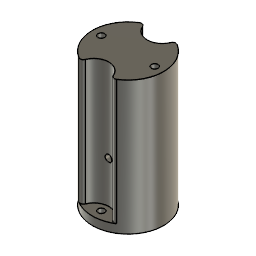
drum (Autodesk Fusion 360 design; units mm, degrees)
part number: 2026-03-23-22-00-02-455
Autodesk Fusion 360 part; units mm, degrees
sketch "Sketch1" plane through (0, 0, 0) normal (0, 0, 1) x (1, 0, 0)
  circle A0 centre (0, 0) radius 10.7
  circle A1 centre (0, 0) radius 4.05
  line L0 (-10, -10) -> (10, 10)
  line L1 (-10, 10) -> (10, -10)
  circle A2 centre (-8, 0) radius 1
  circle A3 centre (-8, 0) radius 2.25
  circle A4 centre (-10.25, 0) radius 4.5
  circle A5 centre (0, -8) radius 1
  circle A6 centre (0, -8) radius 2.25
  circle A7 centre (0, -10.25) radius 4.5
  circle A8 centre (8, 0) radius 2.25
  circle A9 centre (8, 0) radius 1
  circle A10 centre (10.25, 0) radius 4.5
  circle A11 centre (0, 8) radius 1
  circle A12 centre (0, 8) radius 2.25
  circle A13 centre (0, 10.25) radius 4.5
  dimension "d3" = 21.4
  dimension "d4" = 8.1
  dimension "d19" = 2
  constraint concentric A0 A1
  constraint coincident A3 A4.centre
  constraint symmetric L0 A2 A5
  constraint symmetric L0 A3 A6
  constraint symmetric L0 A4 A7
  constraint symmetric L1 A2 A11
  constraint symmetric L1 A3 A12
  constraint symmetric L1 A4 A13
  constraint symmetric L1 A5 A9
  constraint symmetric L1 A6 A8
  constraint symmetric L1 A7 A10
  measures "d3" diameter of A0
  measures "d4" diameter of A1
  measures "d19" diameter of A9
extrude "Extrude1" add sketch "Sketch1" along normal blind 40 contours A8 | A0 A10 | A0 A1 L0 L1 A10 | A0 A1 L0 L1 A13 | A0 A1 L0 L1 A7 | A12 | A0 A13 | A1 L0 L1 | A1 L0 L1 | A6 | A0 A7 | A1 L0 L1 | A1 L0 L1 | A0 A1 L0 L1 A4 | A3 | A0 A4 | A2 | A5 | A9 | A11 picked at (9.1824, 3.0854) picked at (3.1202, 9.1627) picked at (3.1202, -9.1627) picked at (-9.1824, -3.0854)
extrude "Extrude2" cut sketch "Sketch1" along normal blind 2 contours A1 L0 L1 | A1 L0 L1 | A1 L0 L1 | A1 L0 L1
extrude "Extrude3" cut sketch "Sketch1" along normal up to surface (40 mm away) contours A2 | A5 | A9 | A11
extrude "Extrude4" cut sketch "Sketch1" along normal up to surface (37.5 mm away) from surface at 2.5 contours A12 | A0 A13 | A6 | A0 A7 picked at (3.1202, 9.1627) picked at (3.1202, -9.1627)
sketch "Sketch2" plane through (0, 0, 0) normal (0, 1, 0) x (1, 0, 0)
  circle A0 centre (0, -15) radius 1
  line L0 (0, 2.046) -> (0, -15) construction
  dimension "d20" = 17.046
  constraint vertical L0
  constraint coincident A0.centre L0.end
  measures "d20" distance of L0.start A0.centre
extrude "Extrude5" cut sketch "Sketch2" along normal through all and the other way through all
fillet "Fillet1" radius 1 5 edges at (-4.4689, -9.7221, 21.25) (4.4689, -9.7221, 21.25) (-4.4689, -9.7221, 21.25) (4.4689, 9.7221, 21.25) (-4.4689, 9.7221, 21.25)
equation "d20 = ( 34.092 / 2 ) * 1 mm"
